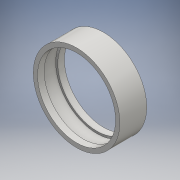
# Autodesk Inventor part: CouplingHead_Silicone
Saved by Autodesk Inventor 2016 (Build 200138000, 138)
## iProperties
Created: 2015-11-25
Part Number: CouplingHead_Silicone
Material: UHMW, White
Document SubType Name: Modeling
Designer: momem
Density: 0.94 g/cm^3
Appearance: Smooth - White
d0: 38.593 mm
d7: 40.593 mm
WoodThickness: 6.390 mm
BearingHolderHeight: 13.100 mm
Author: momem
Autodesk Inventor part; units mm, degrees
ref_plane "YZ Plane" through (0, 0, 0) normal (1, 0, 0) x (0, 1, 0)
ref_plane "XZ Plane" through (0, 0, 0) normal (0, 1, 0) x (-1, 0, 0)
ref_plane "XY Plane" through (0, 0, 0) normal (0, 0, 1) x (1, 0, 0)
sketch "Sketch1" plane through (0, 0, 0) normal (0, 1, 0) x (-1, 0, 0)
  circle A0 centre (0, 0) radius 19.2963
  circle A1 centre (0, 0) radius 20.2963
  dimension "d0" = 38.5926
  dimension "d7" = 40.5926
  constraints: 2 centre point, 2 coincident
  measures "d0" diameter of A0
  measures "d7" diameter of A1
extrude "Extrusion2" add sketch "Sketch1" along normal blind 12.59
sketch "Sketch2" plane through (0, 12.59, 0) normal (0, 1, 0) x (1, 0, 0)
  circle A0 centre (0, 0) radius 19.2963
  circle A1 centre (0, 0) radius 18.2963
  dimension "d12" = 38.5926
  dimension "d13" = 36.5926
  constraints: 2 centre point, 2 coincident
  measures "d12" diameter of A0
  measures "d13" diameter of A1
extrude "Extrusion3" add sketch "Sketch2" against normal blind 3.1
sketch "Sketch3" plane through (0, 0, 0) normal (0, -1, 0) x (1, 0, 0)
  circle A0 centre (0, 0) radius 19.2963
  circle A1 centre (0, 0) radius 18.2963
  dimension "d16" = 38.5926
  dimension "d17" = 36.5926
  constraints: 2 centre point, 2 coincident
  measures "d16" diameter of A0
  measures "d17" diameter of A1
extrude "Extrusion4" add sketch "Sketch3" against normal blind 3.1
equation "\"d7\" = -2 * WoodThickness + 2 * d176 - 2 * d125"
equation "\"d12\" = d0"
equation "\"d16\" = d0"
equation "\"WoodThickness\" = 6.39"
equation "\"BearingHolderHeight\" = 13.1"
equation "\"d176\" = 34.539"
equation "\"d125\" = 7.852683"
body "Solid2"
